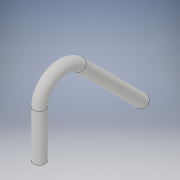
# Autodesk Inventor part: rope hole
Saved by Autodesk Inventor 2019 (Build 230136000, 136)
## iProperties
Created: 2018-09-06
Part Number: rope hole
Material: Generic
Document SubType Name: Modeling
Designer: HIVE
Density: 1 g/cm^3
Appearance: Default
Author: HIVE
## iProperties of the stored document rope hole_3DPrint.ipt
Created: 2018-09-06
Part Number: rope hole_3DPrint
Material: Generic
Document SubType Name: Modeling
Designer: HIVE
Density: 1 g/cm^3
Appearance: Default
Author: HIVE
Autodesk Inventor part; units mm, degrees
ref_plane "YZ Plane" through (0, 0, 0) normal (1, 0, 0) x (0, 1, 0)
ref_plane "XZ Plane" through (0, 0, 0) normal (0, 1, 0) x (-1, 0, 0)
ref_plane "XY Plane" through (0, 0, 0) normal (0, 0, 1) x (1, 0, 0)
sketch "Sketch1" plane through (0, 0, 0) normal (0, 1, 0) x (-1, 0, 0)
  circle A0 centre (0, 0) radius 2.5
  dimension "d0" = 5
  constraints: 1 centre point, 1 coincident
  measures "d0" diameter of A0
sketch "Sketch2" plane through (0, 0, 0) normal (1, 0, 0) x (0, 1, 0)
  line L0 (0, 0) -> (20, 0)
  arc A0 (27.0711, -17.0711) -> (20, 0) centre (20, -10) ccw
  line L1 (0, -53.443) -> (0, 11.6633) projected
  line L2 (0, -44.1421) -> (27.0711, -17.0711)
  dimension "d1" = 20
  dimension "d2" = 10
  dimension "d5" = 45
  constraints: 5 end point, 2 point on circle, 2 tangent, 1 centre point, 1 horizontal, 1 point on line
  measures "d1" distance of L0.start L0.end
  measures "d2" radius of A0
  measures "d5" angle of L1 L2
sweep "Sweep1" add profiles "Sketch1" path "Sketch2" path curves L0 A0 L2
body "Solid1"
